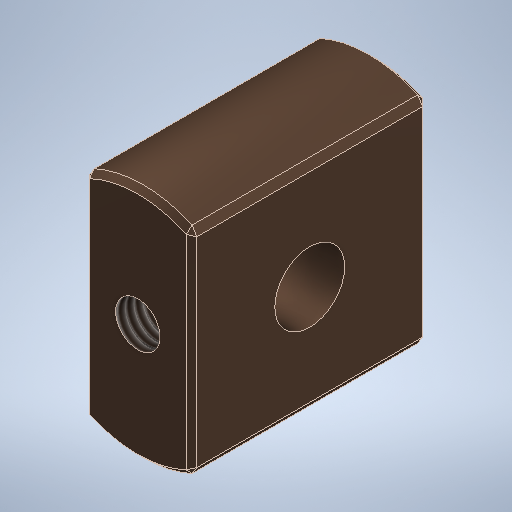
# Autodesk Inventor part: 19 - Crosshead
Saved by Autodesk Inventor 2025.2 (Build 292293000, 293)
## iProperties
Created: 2025-06-19
Part Number: 19 - Crosshead
Material: Bronze, Soft Tin
Document SubType Name: Modeling
Designer: bless
Density: 8.874 g/cm^3
Appearance: Bronze - Satin
Author: bless
Autodesk Inventor part; units mm, degrees
ref_plane "YZ Plane" through (0, 0, 0) normal (1, 0, 0) x (0, 1, 0)
ref_plane "XZ Plane" through (0, 0, 0) normal (0, 1, 0) x (-1, 0, 0)
ref_plane "XY Plane" through (0, 0, 0) normal (0, 0, 1) x (1, 0, 0)
sketch "Sketch1" plane through (0, 0, 0) normal (0, 0, 1) x (1, 0, 0)
  line L0 (5, 9.798) -> (5, -9.798)
  line L1 (-5, -9.798) -> (-5, 9.798)
  arc A0 (-5, -9.798) -> (5, -9.798) centre (0, 0) ccw
  arc A1 (5, 9.798) -> (-5, 9.798) centre (0, 0) ccw
  point P0 (0, 12.4867)
  point P1 (5, 0)
  dimension "d1" = 10
  dimension "d2" = 11
  dimension "d3" = 11
  dimension "d4" = 5
  dimension "d5" = 12.4867
  constraints: 4 end point, 4 point on circle, 2 centre point, 1 coincident, 1 midpoint, 1 parallel, 1 vertical, 1 vertical alignment
  measures "d1" distance between parallel lines of L0 L1
  measures "d2" radius of A1
  measures "d3" radius of A0
  measures "d4" distance of point (0, 0) point (5, 0)
  measures "d5" distance of point (0, 12.487) point (0, 0)
extrude "Extrusion1" add sketch "Sketch1" along normal blind 22
chamfer "Chamfer1" distance 0.5 angle 45 12 edges at (0, 11, 22) (5, 0, 22) (0, -11, 22) (-5, 0, 22) (5, 9.798, 11) (-5, 9.798, 11) (0, 11, 0) (5, 0, 0) (5, -9.798, 11) (0, -11, 0) (-5, 0, 0) (-5, -9.798, 11)
sketch "Sketch2" plane through (0, 0, 22) normal (0, 0, 1) x (1, 0, 0)
  arc A0 (4.5, 9.4868) -> (-4.5, 9.4868) centre (0, 0) ccw projected
  constraints: 1 coincident
hole "Hole1" at (0, 0, 22) direction (0, 0, -1) diameter 4.134 depth 8 thread size "M5x0.8" class "6H" standard "ANSI Metric M Profile"
sketch "Sketch3" plane through (5, -9.298, 0.5) normal (1, 0, 0) x (0, 0, -1)
  line L0 (-21, 18.5959) -> (0, 18.5959) projected
  line L1 (-21, 0) -> (-21, 18.5959) projected
  point P0 (0.5, 9.298)
  point P1 (-10.5, 9.298)
  point P2 (-21, 9.298)
  point P3 (-10.5, 18.5959)
  constraints: 2 midpoint, 1 horizontal alignment, 1 vertical alignment
hole "Hole2" at (5, 0, 11) direction (-1, 0, 0) diameter 6.5 end through all
body "Solid1"
